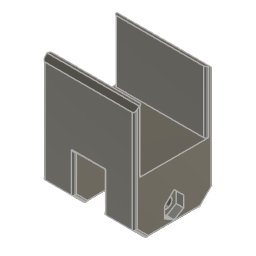
StandingDeskStabilizer (Autodesk Fusion 360 design; units mm, degrees)
Autodesk Fusion 360 part; units mm, degrees
sketch "Sketch1" plane through (0, 0, 0) normal (0, 0, 1) x (1, 0, 0)
  line L0 (18.6, 15.9) -> (-18.6, 15.9)
  line L1 (-18.6, 15.9) -> (-18.6, -15.9)
  line L2 (-18.6, -15.9) -> (18.6, -15.9)
  line L3 (18.6, -15.9) -> (18.6, 15.9)
  line L4 (18.6, 15.9) -> (-18.6, -15.9) construction
  line L5 (-18.6, 15.9) -> (18.6, -15.9) construction
  line L6 (-18.6, -12.9) -> (18.6, -12.9)
  line L7 (-18.6, 12.9) -> (18.6, 12.9)
  line L8 (-5.9, 15.9) -> (-5.9, -15.9)
  line L9 (5.9, 15.9) -> (5.9, -15.9)
  line L10 (0, 0) -> (0, -12.9)
  dimension "d14" = 37.2
  dimension "d15" = 31.8
  dimension "d16" = 3
  dimension "d17" = 3
  dimension "d19" = 11.8
  constraint horizontal L0
  constraint perpendicular L0 L1
  constraint parallel L0 L2
  constraint parallel L1 L3
  constraint coincident L4 L10.start
  constraint coincident L5 L10.start
  constraint coincident L10.start origin
  constraint coincident L1 L6.start
  constraint coincident L3 L6.end
  constraint perpendicular L3 L6
  constraint coincident L1 L7.start
  constraint coincident L3 L7.end
  constraint perpendicular L3 L7
  constraint coincident L0 L8.start
  constraint coincident L2 L8.end
  constraint perpendicular L2 L8
  constraint coincident L0 L9.start
  constraint coincident L2 L9.end
  constraint perpendicular L2 L9
  constraint midpoint L6 L10.end
  constraint symmetric L8 L9 L10
  measures "d14" distance of L1.end L2.end
  measures "d15" distance of L0.end L1.end
  measures "d16" distance of L2 L6
  measures "d17" distance of L0 L7
  measures "d19" distance of L8 L9
extrude "Extrude1" add sketch "Sketch1" along normal blind 3
extrude "Extrude2" add sketch "Sketch1" against normal blind 25 contours L0 L3 L7 L9 | L0 L7 L8 L9 | L0 L1 L7 L8 | L2 L3 L6 L9 | L2 L6 L8 L9 | L1 L2 L6 L8
extrude "Extrude3" add sketch "Sketch1" along normal blind 23 contours L0 L3 L7 L9 | L3 L6 L7 L9 | L0 L1 L7 L8 | L2 L3 L6 L9 | L1 L6 L7 L8 | L1 L2 L6 L8
sketch "Sketch2" plane through (18.6, 0, 0) normal (1, 0, 0) x (0, 1, 0)
  line L0 (12.9, -25) -> (15.9, -25)
  line L1 (-12.9, -25) -> (-12.9, 0)
  line L2 (-12.9, 0) -> (12.9, 0)
  line L3 (12.9, 0) -> (12.9, -25)
  line L4 (15.9, -25) -> (15.9, 23)
  line L5 (15.9, 23) -> (-15.9, 23)
  line L6 (-15.9, 23) -> (-15.9, -25)
  line L7 (0, 0) -> (0, 23) construction
  circle A0 centre (0, 17.3) radius 12.7 construction
  line L8 (-15.9, 0) -> (15.9, 0) construction
  circle A1 centre (0, 17.3) radius 2.15
  circle A2 centre (0, 17.3) radius 4.25
  line L9 (-15.9, -25) -> (-12.9, -25)
  line L10 (-12.7, 17.3) -> (12.7, 17.3) construction
  line L11 (3.0406, 17.3) -> (0, 14.2594)
  line L12 (-3.0406, 17.3) -> (0, 14.2594)
  line L13 (6.0104, 17.3) -> (0, 11.2896)
  line L14 (-6.0104, 17.3) -> (0, 11.2896)
  point P0 (0, 17.3)
  dimension "d29" = 25.4
  dimension "d30" = 17.3
  dimension "d31" = 4.3
  dimension "d32" = 8.5
  constraint coincident L7.start origin
  constraint midpoint L5 L7.end
  constraint coincident L7 P0
  constraint concentric A0 A1
  constraint concentric A1 A2
  constraint coincident P0 A0.centre
  constraint horizontal L10
  constraint coincident P0 L10
  constraint coincident A0 L10.end
  constraint coincident A0 L10.start
  constraint coincident L10 L11.start
  constraint coincident L7 L11.end
  constraint coincident L10 L12.start
  constraint tangent A1 L12
  constraint tangent A1 L11
  constraint perpendicular L11 L12
  constraint coincident L10 L13.start
  constraint coincident L7 L13.end
  constraint coincident L10 L14.start
  constraint tangent A2 L14
  constraint tangent A2 L13
  constraint perpendicular L13 L14
  measures "d29" diameter of A0
  measures "d30" distance of P0 L8
  measures "d31" diameter of A1
  measures "d32" diameter of A2
sketch "Sketch3" plane through (-18.6, 0, 0) normal (-1, 0, 0) x (0, -1, 0)
  line L0 (-15.9, 23) -> (-15.9, -25)
  line L1 (-15.9, -25) -> (-12.9, -25)
  line L2 (-12.9, -25) -> (-12.9, 0)
  line L3 (-12.9, 0) -> (12.9, 0)
  line L4 (12.9, 0) -> (12.9, -25)
  line L5 (12.9, -25) -> (15.9, -25)
  line L6 (15.9, -25) -> (15.9, 23)
  line L7 (15.9, 23) -> (-15.9, 23)
  line L8 (0, 0) -> (0, 17.3) construction
  line L9 (3.85, 15.0772) -> (3.85, 19.5228)
  line L10 (3.85, 19.5228) -> (0, 21.7456)
  line L11 (0, 21.7456) -> (-3.85, 19.5228)
  line L12 (-3.85, 19.5228) -> (-3.85, 15.0772)
  line L13 (-3.85, 15.0772) -> (0, 12.8544) construction
  line L14 (0, 12.8544) -> (3.85, 15.0772) construction
  line L15 (3.85, 15.0772) -> (0, 11.2272)
  line L16 (-3.85, 15.0772) -> (0, 11.2272)
  point P0 (0, 17.3)
  dimension "d45" = 17.3
  dimension "d46" = 3.85
  dimension "d47" = 90
  constraint coincident L8.start origin
  constraint perpendicular L3 L8
  constraint coincident P0 L8.end
  constraint vertical L9
  constraint coincident L8 L15.end
  measures "d45" distance of L8.start P0
  measures "d46" distance of P0 L14
  measures "d47" angle of L15 L16
extrude "Extrude4" cut sketch "Sketch2" against normal up to surface (37.2 mm away) contours A1 | A1 L11 L12
extrude "Extrude5" cut sketch "Sketch2" against normal blind 2.1 contours A1 L11 L12 | A2 | A2 L13 L14
extrude "Extrude7" cut sketch "Sketch3" against normal blind 3 contours L9 L10 L11 L12 L15 L16
chamfer "Chamfer2" distance 5 angle 45 4 edges at (-12.25, -15.9, 23) (12.25, -15.9, 23) (12.25, 15.9, 23) (-12.25, 15.9, 23)
chamfer "Chamfer3" distance 0.78 angle 45 3 edges at (-5.9, 0, 19.45) (-5.9, 0.7601, 15.0196) (-5.9, -0.7601, 15.0196)
chamfer "Chamfer1" distance 1.8 angle 45 2 edges at (0, 15.9, -25) (0, -15.9, -25)
fillet "Fillet1" radius 1 30 edges at (18.6, -15.9, -2.6) (18.6, 15.9, -2.6) (5.9, 15.9, 10.5) (5.9, -15.9, 10.5) (-5.9, -15.9, 10.5) (-5.9, 15.9, 10.5) (-18.6, -15.9, -2.6) (-18.6, 15.9, -2.6) (18.6, -12.9, -12.5) (-18.6, -12.9, -12.5) (18.6, 12.9, -12.5) (-18.6, 12.9, -12.5) (-18.6, 13.4, 20.5) (-5.9, 13.4, 20.5) (5.9, 13.4, 20.5) (18.6, 13.4, 20.5) (18.6, -13.4, 20.5) (5.9, -13.4, 20.5) (-5.9, -13.4, 20.5) (-18.6, -13.4, 20.5) (0, -15.9, 3) (0, 15.9, 3) (12.25, 10.9, 23) (12.25, -10.9, 23) (5.9, 0, 23) (18.6, 0, 23) (-18.6, 0, 23) (-12.25, -10.9, 23) (-5.9, 0, 23) (-12.25, 10.9, 23)
move_body "Move1" bodies 1 to x (-1, 0, 0) y (0, 1, 0) z (0, 0, -1) at (0, 0, 6)
equation "DeskThickness = 25 mm"
equation "PrinterTolerance = 0.4 mm"
equation "DeskAttachmentThickness = 3 mm"
equation "DeskAttachmentDepth = 25 mm"
equation "ScrewTotalWidth = 37.2 mm"
equation "WheelThickness = 11 mm"
equation "WheelDiameter = 25 mm"
equation "ScrewDiameter = 3.9 mm"
equation "ScrewHeadDiameter = 8.1 mm"
equation "ScrewHeadLength = 2.1 mm"
equation "ScrewNutThickness = 3 mm"
equation "ScrewNutCircumscribedDiameter = 6.9 mm"
equation "d14 = ScrewTotalWidth"
equation "d15 = DeskThickness + 2 * DeskAttachmentThickness + 2 * PrinterTolerance"
equation "d16 = DeskAttachmentThickness"
equation "d17 = DeskAttachmentThickness"
equation "d19 = WheelThickness + 2 * PrinterTolerance"
equation "StabilizerCoreThickness = DeskAttachmentThickness" comment "Hex screw distance between parallel sides"
equation "d21 = StabilizerCoreThickness"
equation "d23 = -DeskAttachmentDepth"
equation "d25 = DeskAttachmentThickness - PrinterTolerance * 3"
equation "d27 = 0.8 * WheelDiameter + StabilizerCoreThickness"
equation "d29 = WheelDiameter + PrinterTolerance"
equation "d30 = ( WheelDiameter / 2 ) + StabilizerCoreThickness + 2 * PrinterTolerance + 1 mm"
equation "d31 = ScrewDiameter + PrinterTolerance"
equation "d32 = ScrewHeadDiameter + PrinterTolerance"
equation "d35 = -ScrewHeadLength"
equation "d41 = WheelDiameter / 5"
equation "d42 = ScrewDiameter / 5"
equation "d45 = ( WheelDiameter / 2 ) + StabilizerCoreThickness + 2 * PrinterTolerance + 1 mm"
equation "d46 = ScrewNutCircumscribedDiameter / 2 + PrinterTolerance"
equation "d48 = -ScrewNutThickness"
